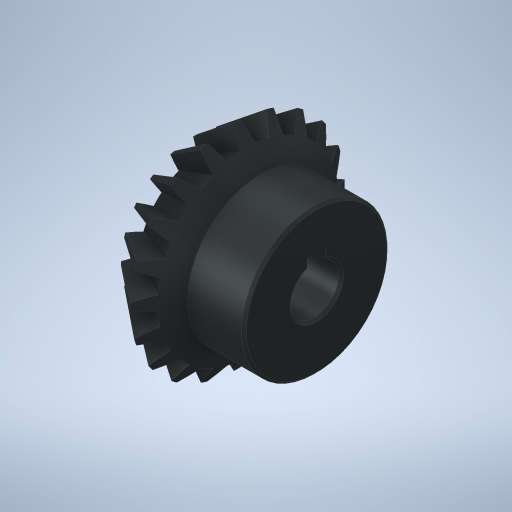
# Autodesk Inventor part: SB2-2030_On
Saved by Autodesk Inventor 2023 (Build 270158000, 158)
## iProperties
Category: PARTsolutions
Company: KHK
Created: 2023-07-20
Part Number: SB2-2030_On
Material: Iron, Cast
Catalog Web Link: www.cadenas.de
Description: Bevel Gears (SB)-L-
Vendor: KHK
Document SubType Name: Modeling
Designer: psAdmin
Manufacturer: KHK
Mass: 119.753 g
Surface Area: 60.1568 cm^2
Volume: 16.7487 cm^3
Density: 7.15 g/cm^3
Appearance: Iron Gray
PSOL_IDENT_0: {$CADENAS_DATA/23d-libs/khk/bevel_gears/sb_l.prj},178 {VTYP=3D},{NB=SB2-2030_On},{LINA=SB2-2030},{NN=
PSOL_IDENT_1: Bevel Gears (SB)-L},{DATE=06.10.2022 23:14:39},{GEOMDATE=08.01.2020 08:57:38},{VERSION=},{LINEID=144
PSOL_IDENT_2: 0},{WBVAR=TOOTH},{WBNUMERIC=}  {NB=SB2-2030_On},{LINA=SB2-2030},{KT=DUMMY},{CN=SB2-2030},{M=2.0},{Z=
PSOL_IDENT_3: 20},{A=10},{B=30},{C=40.0},{D=44.18},{E=45},{F=25.06},{G=16.39},{H=11.67},{I=22.0},{J=11},{K=21.34},
PSOL_IDENT_4: {L=38.27},{S=B3},{PN=SB2-3020},{WMF=B3010.WMF},{X=0.5},{Y=0.5},{R=0.0},{H1=0.00},{VERS=2},{I1=0},{I2=
PSOL_IDENT_5: 0},{AN=0},{H11=0},{TOOTH=On},{ANGLE=48.000},{ANGLE2=0.700}
NB: SB2-2030_On
NN: Bevel Gears (SB)-L
NBSYN: $CN._$TOOTH.
LINA: SB2-2030
CATALOG: KHK
CN: SB2-2030
M: 2
Z: 20
A: 10
B: 30
C: 40
D: 44.18
E: 45
F: 25.06
G: 16.39
H: 11.67
I: 22
J: 11
K: 21.34
L: 38.27
S: B3
PN: SB2-3020
WMF: B3010.WMF
X: 0.5
Y: 0.5
R: 0
H1: 0
VERS: 2
I1: 0
I2: 0
AN: 0
H11: 0
TOOTH: On
ANGLE: 48
ANGLE2: 0.7
SUPPLIER: KHK
ARTICLENO: SB2-2030_On
BOMINFO: SB2-2030
CREATOR: CADENAS GmbH
Title: SB2-2030
Author: Cadenas PARTsolutions
Autodesk Inventor part; units mm, degrees
ref_plane "YZ Plane" through (0, 0, 0) normal (1, 0, 0) x (0, 1, 0)
ref_plane "XZ Plane" through (0, 0, 0) normal (0, 1, 0) x (-1, 0, 0)
ref_plane "XY Plane" through (0, 0, 0) normal (0, 0, 1) x (1, 0, 0)
sketch "Sketch_4" plane through (33.33, 0, 0) normal (-1, 0, 0) x (0, 0, -1)
  arc A0 (-0.6689, 26.6095) -> (-1.7638, 15.9762) centre (40.0225, 17.0467) ccw
  arc A1 (-1.7638, 15.9762) -> (-3.2594, 15.7393) centre (0, 0) ccw
  arc A2 (-3.2594, 15.7393) -> (-7.5866, 25.5139) centre (-43.3314, 3.8447) ccw
  arc A3 (-7.5866, 25.5139) -> (-8.859, 25.1005) centre (0, 0) ccw
  arc A4 (-8.859, 25.1005) -> (-6.6144, 14.6492) centre (32.796, 28.58) ccw
  arc A5 (-6.6144, 14.6492) -> (-7.9636, 13.9617) centre (0, 0) ccw
  arc A6 (-7.9636, 13.9617) -> (-15.0995, 21.9207) centre (-42.3987, -9.7336) ccw
  arc A7 (-15.0995, 21.9207) -> (-16.1819, 21.1344) centre (0, 0) ccw
  arc A8 (-16.1819, 21.1344) -> (-10.8175, 11.8883) centre (22.3591, 37.3157) ccw
  arc A9 (-10.8175, 11.8883) -> (-11.8883, 10.8175) centre (0, 0) ccw
  arc A10 (-11.8883, 10.8175) -> (-21.1344, 16.1819) centre (-37.3157, -22.3591) ccw
  arc A11 (-21.1344, 16.1819) -> (-21.9207, 15.0995) centre (0, 0) ccw
  arc A12 (-21.9207, 15.0995) -> (-13.9617, 7.9636) centre (9.7336, 42.3987) ccw
  arc A13 (-13.9617, 7.9636) -> (-14.6492, 6.6144) centre (0, 0) ccw
  arc A14 (-14.6492, 6.6144) -> (-25.1005, 8.859) centre (-28.58, -32.796) ccw
  arc A15 (-25.1005, 8.859) -> (-25.5139, 7.5866) centre (0, 0) ccw
  arc A16 (-25.5139, 7.5866) -> (-15.7393, 3.2594) centre (-3.8447, 43.3314) ccw
  arc A17 (-15.7393, 3.2594) -> (-15.9762, 1.7638) centre (0, 0) ccw
  arc A18 (-15.9762, 1.7638) -> (-26.6095, 0.6689) centre (-17.0467, -40.0225) ccw
  arc A19 (-26.6095, 0.6689) -> (-26.6095, -0.6689) centre (0, 0) ccw
  arc A20 (-26.6095, -0.6689) -> (-15.9762, -1.7638) centre (-17.0467, 40.0225) ccw
  arc A21 (-15.9762, -1.7638) -> (-15.7393, -3.2594) centre (0, 0) ccw
  arc A22 (-15.7393, -3.2594) -> (-25.5139, -7.5866) centre (-3.8447, -43.3314) ccw
  arc A23 (-25.5139, -7.5866) -> (-25.1005, -8.859) centre (0, 0) ccw
  arc A24 (-25.1005, -8.859) -> (-14.6492, -6.6144) centre (-28.58, 32.796) ccw
  arc A25 (-14.6492, -6.6144) -> (-13.9617, -7.9636) centre (0, 0) ccw
  arc A26 (-13.9617, -7.9636) -> (-21.9207, -15.0995) centre (9.7336, -42.3987) ccw
  arc A27 (-21.9207, -15.0995) -> (-21.1344, -16.1819) centre (0, 0) ccw
  arc A28 (-21.1344, -16.1819) -> (-11.8883, -10.8175) centre (-37.3157, 22.3591) ccw
  arc A29 (-11.8883, -10.8175) -> (-10.8175, -11.8883) centre (0, 0) ccw
  arc A30 (-10.8175, -11.8883) -> (-16.1819, -21.1344) centre (22.3591, -37.3157) ccw
  arc A31 (-16.1819, -21.1344) -> (-15.0995, -21.9207) centre (0, 0) ccw
  arc A32 (-15.0995, -21.9207) -> (-7.9636, -13.9617) centre (-42.3987, 9.7336) ccw
  arc A33 (-7.9636, -13.9617) -> (-6.6144, -14.6492) centre (0, 0) ccw
  arc A34 (-6.6144, -14.6492) -> (-8.859, -25.1005) centre (32.796, -28.58) ccw
  arc A35 (-8.859, -25.1005) -> (-7.5866, -25.5139) centre (0, 0) ccw
  arc A36 (-7.5866, -25.5139) -> (-3.2594, -15.7393) centre (-43.3314, -3.8447) ccw
  arc A37 (-3.2594, -15.7393) -> (-1.7638, -15.9762) centre (0, 0) ccw
  arc A38 (-1.7638, -15.9762) -> (-0.6689, -26.6095) centre (40.0225, -17.0467) ccw
  arc A39 (-0.6689, -26.6095) -> (0.6689, -26.6095) centre (0, 0) ccw
  arc A40 (0.6689, -26.6095) -> (1.7638, -15.9762) centre (-40.0225, -17.0467) ccw
  arc A41 (1.7638, -15.9762) -> (3.2594, -15.7393) centre (0, 0) ccw
  arc A42 (3.2594, -15.7393) -> (7.5866, -25.5139) centre (43.3314, -3.8447) ccw
  arc A43 (7.5866, -25.5139) -> (8.859, -25.1005) centre (0, 0) ccw
  arc A44 (8.859, -25.1005) -> (6.6144, -14.6492) centre (-32.796, -28.58) ccw
  arc A45 (6.6144, -14.6492) -> (7.9636, -13.9617) centre (0, 0) ccw
  arc A46 (7.9636, -13.9617) -> (15.0995, -21.9207) centre (42.3987, 9.7336) ccw
  arc A47 (15.0995, -21.9207) -> (16.1819, -21.1344) centre (0, 0) ccw
  arc A48 (16.1819, -21.1344) -> (10.8175, -11.8883) centre (-22.3591, -37.3157) ccw
  arc A49 (10.8175, -11.8883) -> (11.8883, -10.8175) centre (0, 0) ccw
  arc A50 (11.8883, -10.8175) -> (21.1344, -16.1819) centre (37.3157, 22.3591) ccw
  arc A51 (21.1344, -16.1819) -> (21.9207, -15.0995) centre (0, 0) ccw
  arc A52 (21.9207, -15.0995) -> (13.9617, -7.9636) centre (-9.7336, -42.3987) ccw
  arc A53 (13.9617, -7.9636) -> (14.6492, -6.6144) centre (0, 0) ccw
  arc A54 (14.6492, -6.6144) -> (25.1005, -8.859) centre (28.58, 32.796) ccw
  arc A55 (25.1005, -8.859) -> (25.5139, -7.5866) centre (0, 0) ccw
  arc A56 (25.5139, -7.5866) -> (15.7393, -3.2594) centre (3.8447, -43.3314) ccw
  arc A57 (15.7393, -3.2594) -> (15.9762, -1.7638) centre (0, 0) ccw
  arc A58 (15.9762, -1.7638) -> (26.6095, -0.6689) centre (17.0467, 40.0225) ccw
  arc A59 (26.6095, -0.6689) -> (26.6095, 0.6689) centre (0, 0) ccw
  arc A60 (26.6095, 0.6689) -> (15.9762, 1.7638) centre (17.0467, -40.0225) ccw
  arc A61 (15.9762, 1.7638) -> (15.7393, 3.2594) centre (0, 0) ccw
  arc A62 (15.7393, 3.2594) -> (25.5139, 7.5866) centre (3.8447, 43.3314) ccw
  arc A63 (25.5139, 7.5866) -> (25.1005, 8.859) centre (0, 0) ccw
  arc A64 (25.1005, 8.859) -> (14.6492, 6.6144) centre (28.58, -32.796) ccw
  arc A65 (14.6492, 6.6144) -> (13.9617, 7.9636) centre (0, 0) ccw
  arc A66 (13.9617, 7.9636) -> (21.9207, 15.0995) centre (-9.7336, 42.3987) ccw
  arc A67 (21.9207, 15.0995) -> (21.1344, 16.1819) centre (0, 0) ccw
  arc A68 (21.1344, 16.1819) -> (11.8883, 10.8175) centre (37.3157, -22.3591) ccw
  arc A69 (11.8883, 10.8175) -> (10.8175, 11.8883) centre (0, 0) ccw
  arc A70 (10.8175, 11.8883) -> (16.1819, 21.1344) centre (-22.3591, 37.3157) ccw
  arc A71 (16.1819, 21.1344) -> (15.0995, 21.9207) centre (0, 0) ccw
  arc A72 (15.0995, 21.9207) -> (7.9636, 13.9617) centre (42.3987, -9.7336) ccw
  arc A73 (7.9636, 13.9617) -> (6.6144, 14.6492) centre (0, 0) ccw
  arc A74 (6.6144, 14.6492) -> (8.859, 25.1005) centre (-32.796, 28.58) ccw
  arc A75 (8.859, 25.1005) -> (7.5866, 25.5139) centre (0, 0) ccw
  arc A76 (7.5866, 25.5139) -> (3.2594, 15.7393) centre (43.3314, 3.8447) ccw
  arc A77 (3.2594, 15.7393) -> (1.7638, 15.9762) centre (0, 0) ccw
  arc A78 (1.7638, 15.9762) -> (0.6689, 26.6095) centre (-40.0225, 17.0467) ccw
  arc A79 (0.6689, 26.6095) -> (-0.6689, 26.6095) centre (0, 0) ccw
  constraints: 160 point on circle, 80 centre point
sketch "Sketch_5" plane through (19.94, 0, 0) normal (-1, 0, 0) x (0, 0, -1)
  arc A0 (-0.2985, 15.8348) -> (-0.9582, 8.6794) centre (40.8411, 8.4338) ccw
  arc A1 (-0.9582, 8.6794) -> (-1.7708, 8.5507) centre (0, 0) ccw
  arc A2 (-1.7708, 8.5507) -> (-4.6093, 15.152) centre (-41.4484, -4.5995) ccw
  arc A3 (-4.6093, 15.152) -> (-5.1771, 14.9676) centre (0, 0) ccw
  arc A4 (-5.1771, 14.9676) -> (-3.5934, 7.9585) centre (36.236, 20.6416) ccw
  arc A5 (-3.5934, 7.9585) -> (-4.3264, 7.585) centre (0, 0) ccw
  arc A6 (-4.3264, 7.585) -> (-9.066, 12.9861) centre (-37.9984, -17.1827) ccw
  arc A7 (-9.066, 12.9861) -> (-9.549, 12.6352) centre (0, 0) ccw
  arc A8 (-9.549, 12.6352) -> (-5.8768, 6.4585) centre (28.0838, 30.8289) ccw
  arc A9 (-5.8768, 6.4585) -> (-6.4585, 5.8768) centre (0, 0) ccw
  arc A10 (-6.4585, 5.8768) -> (-12.6352, 9.549) centre (-30.8289, -28.0838) ccw
  arc A11 (-12.6352, 9.549) -> (-12.9861, 9.066) centre (0, 0) ccw
  arc A12 (-12.9861, 9.066) -> (-7.585, 4.3264) centre (17.1827, 37.9984) ccw
  arc A13 (-7.585, 4.3264) -> (-7.9585, 3.5934) centre (0, 0) ccw
  arc A14 (-7.9585, 3.5934) -> (-14.9676, 5.1771) centre (-20.6416, -36.236) ccw
  arc A15 (-14.9676, 5.1771) -> (-15.152, 4.6093) centre (0, 0) ccw
  arc A16 (-15.152, 4.6093) -> (-8.5507, 1.7708) centre (4.5995, 41.4484) ccw
  arc A17 (-8.5507, 1.7708) -> (-8.6794, 0.9582) centre (0, 0) ccw
  arc A18 (-8.6794, 0.9582) -> (-15.8348, 0.2985) centre (-8.4338, -40.8411) ccw
  arc A19 (-15.8348, 0.2985) -> (-15.8348, -0.2985) centre (0, 0) ccw
  arc A20 (-15.8348, -0.2985) -> (-8.6794, -0.9582) centre (-8.4338, 40.8411) ccw
  arc A21 (-8.6794, -0.9582) -> (-8.5507, -1.7708) centre (0, 0) ccw
  arc A22 (-8.5507, -1.7708) -> (-15.152, -4.6093) centre (4.5995, -41.4484) ccw
  arc A23 (-15.152, -4.6093) -> (-14.9676, -5.1771) centre (0, 0) ccw
  arc A24 (-14.9676, -5.1771) -> (-7.9585, -3.5934) centre (-20.6416, 36.236) ccw
  arc A25 (-7.9585, -3.5934) -> (-7.585, -4.3264) centre (0, 0) ccw
  arc A26 (-7.585, -4.3264) -> (-12.9861, -9.066) centre (17.1827, -37.9984) ccw
  arc A27 (-12.9861, -9.066) -> (-12.6352, -9.549) centre (0, 0) ccw
  arc A28 (-12.6352, -9.549) -> (-6.4585, -5.8768) centre (-30.8289, 28.0838) ccw
  arc A29 (-6.4585, -5.8768) -> (-5.8768, -6.4585) centre (0, 0) ccw
  arc A30 (-5.8768, -6.4585) -> (-9.549, -12.6352) centre (28.0838, -30.8289) ccw
  arc A31 (-9.549, -12.6352) -> (-9.066, -12.9861) centre (0, 0) ccw
  arc A32 (-9.066, -12.9861) -> (-4.3264, -7.585) centre (-37.9984, 17.1827) ccw
  arc A33 (-4.3264, -7.585) -> (-3.5934, -7.9585) centre (0, 0) ccw
  arc A34 (-3.5934, -7.9585) -> (-5.1771, -14.9676) centre (36.236, -20.6416) ccw
  arc A35 (-5.1771, -14.9676) -> (-4.6093, -15.152) centre (0, 0) ccw
  arc A36 (-4.6093, -15.152) -> (-1.7708, -8.5507) centre (-41.4484, 4.5995) ccw
  arc A37 (-1.7708, -8.5507) -> (-0.9582, -8.6794) centre (0, 0) ccw
  arc A38 (-0.9582, -8.6794) -> (-0.2985, -15.8348) centre (40.8411, -8.4338) ccw
  arc A39 (-0.2985, -15.8348) -> (0.2985, -15.8348) centre (0, 0) ccw
  arc A40 (0.2985, -15.8348) -> (0.9582, -8.6794) centre (-40.8411, -8.4338) ccw
  arc A41 (0.9582, -8.6794) -> (1.7708, -8.5507) centre (0, 0) ccw
  arc A42 (1.7708, -8.5507) -> (4.6093, -15.152) centre (41.4484, 4.5995) ccw
  arc A43 (4.6093, -15.152) -> (5.1771, -14.9676) centre (0, 0) ccw
  arc A44 (5.1771, -14.9676) -> (3.5934, -7.9585) centre (-36.236, -20.6416) ccw
  arc A45 (3.5934, -7.9585) -> (4.3264, -7.585) centre (0, 0) ccw
  arc A46 (4.3264, -7.585) -> (9.066, -12.9861) centre (37.9984, 17.1827) ccw
  arc A47 (9.066, -12.9861) -> (9.549, -12.6352) centre (0, 0) ccw
  arc A48 (9.549, -12.6352) -> (5.8768, -6.4585) centre (-28.0838, -30.8289) ccw
  arc A49 (5.8768, -6.4585) -> (6.4585, -5.8768) centre (0, 0) ccw
  arc A50 (6.4585, -5.8768) -> (12.6352, -9.549) centre (30.8289, 28.0838) ccw
  arc A51 (12.6352, -9.549) -> (12.9861, -9.066) centre (0, 0) ccw
  arc A52 (12.9861, -9.066) -> (7.585, -4.3264) centre (-17.1827, -37.9984) ccw
  arc A53 (7.585, -4.3264) -> (7.9585, -3.5934) centre (0, 0) ccw
  arc A54 (7.9585, -3.5934) -> (14.9676, -5.1771) centre (20.6416, 36.236) ccw
  arc A55 (14.9676, -5.1771) -> (15.152, -4.6093) centre (0, 0) ccw
  arc A56 (15.152, -4.6093) -> (8.5507, -1.7708) centre (-4.5995, -41.4484) ccw
  arc A57 (8.5507, -1.7708) -> (8.6794, -0.9582) centre (0, 0) ccw
  arc A58 (8.6794, -0.9582) -> (15.8348, -0.2985) centre (8.4338, 40.8411) ccw
  arc A59 (15.8348, -0.2985) -> (15.8348, 0.2985) centre (0, 0) ccw
  arc A60 (15.8348, 0.2985) -> (8.6794, 0.9582) centre (8.4338, -40.8411) ccw
  arc A61 (8.6794, 0.9582) -> (8.5507, 1.7708) centre (0, 0) ccw
  arc A62 (8.5507, 1.7708) -> (15.152, 4.6093) centre (-4.5995, 41.4484) ccw
  arc A63 (15.152, 4.6093) -> (14.9676, 5.1771) centre (0, 0) ccw
  arc A64 (14.9676, 5.1771) -> (7.9585, 3.5934) centre (20.6416, -36.236) ccw
  arc A65 (7.9585, 3.5934) -> (7.585, 4.3264) centre (0, 0) ccw
  arc A66 (7.585, 4.3264) -> (12.9861, 9.066) centre (-17.1827, 37.9984) ccw
  arc A67 (12.9861, 9.066) -> (12.6352, 9.549) centre (0, 0) ccw
  arc A68 (12.6352, 9.549) -> (6.4585, 5.8768) centre (30.8289, -28.0838) ccw
  arc A69 (6.4585, 5.8768) -> (5.8768, 6.4585) centre (0, 0) ccw
  arc A70 (5.8768, 6.4585) -> (9.549, 12.6352) centre (-28.0838, 30.8289) ccw
  arc A71 (9.549, 12.6352) -> (9.066, 12.9861) centre (0, 0) ccw
  arc A72 (9.066, 12.9861) -> (4.3264, 7.585) centre (37.9984, -17.1827) ccw
  arc A73 (4.3264, 7.585) -> (3.5934, 7.9585) centre (0, 0) ccw
  arc A74 (3.5934, 7.9585) -> (5.1771, 14.9676) centre (-36.236, 20.6416) ccw
  arc A75 (5.1771, 14.9676) -> (4.6093, 15.152) centre (0, 0) ccw
  arc A76 (4.6093, 15.152) -> (1.7708, 8.5507) centre (41.4484, -4.5995) ccw
  arc A77 (1.7708, 8.5507) -> (0.9582, 8.6794) centre (0, 0) ccw
  arc A78 (0.9582, 8.6794) -> (0.2985, 15.8348) centre (-40.8411, 8.4338) ccw
  arc A79 (0.2985, 15.8348) -> (-0.2985, 15.8348) centre (0, 0) ccw
  constraints: 160 point on circle, 80 centre point
loft "Loft1" add profiles "Sketch_4", "Sketch_5"
sketch "Sketch_6" plane through (0, 0, 0) normal (0, 0, 1) x (1, 0, 0)
  line L0 (45, 0) -> (19.94, 0)
  line L1 (23, 0) -> (23, 10.67)
  line L2 (23, 10.67) -> (21.4084, 13.0523)
  line L3 (21.4084, 13.0523) -> (30.9025, 18.6464)
  line L4 (30.9025, 18.6464) -> (33.33, 15)
  line L5 (33.33, 15) -> (44.5, 15)
  line L6 (44.5, 15) -> (45, 14.5)
  line L7 (45, 14.5) -> (45, 0)
  line L8 (45, 0) -> (23, 0)
  constraints: 18 end point
revolve "Revolution1" add sketch "Sketch_6" angle 360 about axis through (45, 0, 0) along (1, 0, 0)
sketch "Sketch_7" plane through (0, 0, 0) normal (0, 0, 1) x (1, 0, 0)
  line L0 (45, 0) -> (0, 0)
  line L1 (0, 0) -> (0, 44.18)
  line L2 (0, 44.18) -> (33.33, 44.18)
  line L3 (33.33, 44.18) -> (33.33, 15)
  line L4 (33.33, 15) -> (28.61, 22.09)
  line L5 (28.61, 22.09) -> (19.94, 15.2502)
  line L6 (19.94, 15.2502) -> (23, 10.67)
  line L7 (23, 10.67) -> (23, 5.5)
  line L8 (23, 5.5) -> (23.5, 5)
  line L9 (23.5, 5) -> (44.5, 5)
  line L10 (44.5, 5) -> (45, 5.5)
  line L11 (45, 5.5) -> (45, 0)
  line L12 (45, 0) -> (0, 0)
  constraints: 26 end point
revolve "Revolution2" cut sketch "Sketch_7" angle 360 about axis through (45, 0, 0) along (1, 0, 0)
ref_plane "IP2_XY" through (0, 0, 0) normal (1, 0, 0) x (0, 0, -1)
ref_plane "IP2_YZ" through (0, 0, 0) normal (0, 0, -1) x (0, 1, 0)
ref_plane "IP2_ZX" through (0, 0, 0) normal (0, 1, 0) x (1, 0, 0)
ref_plane "l_XY" through (0, 0, 0) normal (0, 1, 0) x (1, 0, 0)
ref_plane "l_YZ" through (0, 0, 0) normal (1, 0, 0) x (0, 0, -1)
ref_plane "l_ZX" through (0, 0, 0) normal (0, 0, -1) x (0, 1, 0)
sketch "Sketch5" plane through (45, 0, 0) normal (1, 0, 0) x (0, 0, -1)
  line L0 (-2, 3.2) -> (2, 3.2)
  line L1 (2, 3.2) -> (2, 6.8)
  line L2 (2, 6.8) -> (-2, 6.8)
  line L3 (-2, 6.8) -> (-2, 3.2)
  circle A0 centre (0, 0) radius 5 projected
  line L4 (-2, 3.2) -> (2, 6.8) construction
  line L5 (2, 3.2) -> (-2, 6.8) construction
  point P0 (0, 5)
  dimension "d6" = 4
  dimension "d7" = 1.8
  constraints: 12 end point, 2 midpoint, 2 parallel, 2 vertical alignment, 1 horizontal, 1 perpendicular, 1 other
  measures "d6" distance of L1.end L2.end
  measures "d7" distance from line of point (0, 5) L2
extrude "Extrusion1" cut sketch "Sketch5" against normal through all contours L3 A0 L1 L0 | L3 L2 L1 A0 picked at (0, 3.8)
body "Solid1"
